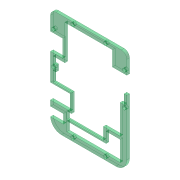
# Autodesk Inventor part: beagle_spacer_top
Saved by Autodesk Inventor 2014 (Build 180170000, 170)
## iProperties
Created: 2013-06-20
Part Number: beagle_spacer_top
Document SubType Name: Modeling
Designer: Administrator
Density: 1 g/cm^3
Mass: 28.363 g
Surface Area: 163.397 cm^2
Volume: 28.363 cm^3
Material: Generic
Appearance: Clear - Green 1
Author: Administrator
Autodesk Inventor part; units mm, degrees
ref_plane "YZ Plane" through (0, 0, 0) normal (1, 0, 0) x (0, 1, 0)
ref_plane "XZ Plane" through (0, 0, 0) normal (0, 1, 0) x (-1, 0, 0)
ref_plane "XY Plane" through (0, 0, 0) normal (0, 0, 1) x (1, 0, 0)
sketch "Sketch1" plane through (0, 0, 0) normal (0, 0, 1) x (1, 0, 0)
  line L0 (9.8795, 48.1994) -> (9.8795, -53.4006)
  line L1 (16.2295, 54.5494) -> (92.4295, 54.5494)
  line L2 (98.7795, 48.1994) -> (98.7795, -53.4006)
  line L3 (22.5795, -66.1006) -> (86.0795, -66.1006)
  arc A0 (9.8795, -53.4006) -> (22.5795, -66.1006) centre (22.5795, -53.4006) ccw
  arc A1 (16.2295, 54.5494) -> (9.8795, 48.1994) centre (16.2295, 48.1994) ccw
  arc A2 (98.7795, 48.1994) -> (92.4295, 54.5494) centre (92.4295, 48.1994) ccw
  arc A3 (86.0795, -66.1006) -> (98.7795, -53.4006) centre (86.0795, -53.4006) ccw
  point P0 (0, 0)
  dimension "d0" = 12.7
  dimension "d1" = 6.35
  dimension "d2" = 120.65
  dimension "d3" = 88.9
  constraints: 8 end point, 8 point on circle, 8 tangent, 4 centre point, 2 equal radius, 1 horizontal, 1 vertical
  measures "d0" radius of A0
  measures "d1" radius of A1
  measures "d2" distance between parallel lines of L3 L1
  measures "d3" distance between parallel lines of L2 L0
extrude "Extrusion1" add sketch "Sketch1" along normal blind 3.175
sketch "Sketch2" plane through (0, 0, 3.175) normal (0, 0, 1) x (1, 0, 0)
  line L0 (9.8795, -53.4006) -> (9.8795, 48.1994) projected
  line L1 (98.7795, 48.1994) -> (98.7795, -53.4006) projected
  line L2 (16.2295, 54.5494) -> (92.4295, 54.5494) projected
  line L3 (26.6435, 49.4694) -> (82.0155, 49.4694)
  line L4 (82.0155, 49.4694) -> (82.0155, -1.3306)
  line L5 (82.0155, -1.3306) -> (26.6435, -1.3306)
  line L6 (26.6435, -1.3306) -> (26.6435, 49.4694)
  point P0 (0, 0)
  dimension "d13" = 16.764
  dimension "d14" = 16.764
  dimension "d15" = 5.08
  dimension "d16" = 55.88
  constraints: 8 end point
  measures "d13" distance between parallel lines of L0 L6
  measures "d14" distance between parallel lines of L1 L4
  measures "d15" distance between parallel lines of L2 L3
  measures "d16" distance between parallel lines of L5 L2
extrude "Extrusion2" cut sketch "Sketch2" against normal through all
sketch "Sketch3" plane through (0, 0, 3.175) normal (0, 0, 1) x (1, 0, 0)
  line L0 (9.8795, -53.4006) -> (9.8795, 48.1994) projected
  line L1 (86.0795, -66.1006) -> (22.5795, -66.1006) projected
  line L2 (9.8795, -19.4408) -> (32.7395, -19.4408)
  line L3 (32.7395, -19.4408) -> (32.7395, -37.2208)
  line L4 (32.7395, -37.2208) -> (9.8795, -37.2208)
  point P0 (0, 0)
  dimension "d20" = 28.8798
  dimension "d21" = 46.6598
  dimension "d22" = 22.86
  constraints: 6 end point, 2 point on line
  measures "d20" distance between parallel lines of L4 L1
  measures "d21" distance between parallel lines of L1 L2
  measures "d22" distance between parallel lines of L3 L0
extrude "Extrusion3" cut sketch "Sketch3" against normal through all
sketch "Sketch4" plane through (0, 0, 3.175) normal (0, 0, 1) x (1, 0, 0)
  line L0 (9.8795, -53.4006) -> (9.8795, -37.2208) projected
  arc A0 (9.8795, -53.4006) -> (22.5795, -66.1006) centre (22.5795, -53.4006) ccw projected
  line L1 (86.0795, -66.1006) -> (22.5795, -66.1006) projected
  line L2 (24.8655, -43.5708) -> (24.8655, -54.1626)
  line L3 (24.8655, -43.5708) -> (9.8795, -43.5708)
  line L4 (24.8655, -54.1626) -> (9.9024, -54.1626)
  point P0 (0, 0)
  dimension "d26" = 22.5298
  dimension "d27" = 14.986
  dimension "d28" = 11.938
  constraints: 6 end point, 1 horizontal, 1 point on circle, 1 point on line, 1 vertical
  measures "d26" distance between parallel lines of L1 L3
  measures "d27" distance between parallel lines of L0 L2
  measures "d28" distance between parallel lines of L1 L4
extrude "Extrusion4" cut sketch "Sketch4" against normal through all
sketch "Sketch5" plane through (0, 0, 3.175) normal (0, 0, 1) x (1, 0, 0)
  line L0 (86.0795, -66.1006) -> (22.5795, -66.1006) projected
  line L1 (9.8795, -19.4408) -> (9.8795, 48.1994) projected
  line L2 (9.8795, -43.5708) -> (9.8795, -37.2208) projected
  line L3 (28.9295, -2.1688) -> (91.1595, -2.1688)
  line L4 (91.1595, -2.1688) -> (91.1595, -11.5668)
  line L5 (91.1595, -11.5668) -> (28.9295, -11.5668)
  line L6 (28.9295, -11.5668) -> (28.9295, -2.1688)
  line L7 (28.9295, -50.4288) -> (91.1595, -50.4288)
  line L8 (91.1595, -50.4288) -> (91.1595, -59.8268)
  line L9 (91.1595, -59.8268) -> (28.9295, -59.8268)
  line L10 (28.9295, -59.8268) -> (28.9295, -50.4288)
  point P0 (0, 0)
  dimension "d31" = 54.5338
  dimension "d32" = 9.398
  dimension "d33" = 62.23
  dimension "d34" = 19.05
  dimension "d35" = 19.05
  dimension "d36" = 6.2738
  constraints: 16 end point, 2 equal length
  measures "d31" distance between parallel lines of L0 L5
  measures "d32" distance between parallel lines of L3 L5
  measures "d33" distance of L4.end L5.end
  measures "d34" distance between parallel lines of L1 L6
  measures "d35" distance between parallel lines of L2 L10
  measures "d36" distance between parallel lines of L9 L0
extrude "Extrusion5" cut sketch "Sketch5" against normal through all
sketch "Sketch6" plane through (0, 0, 3.175) normal (0, 0, 1) x (1, 0, 0)
  line L0 (74.6495, -11.5668) -> (28.9295, -11.5668)
  line L1 (28.9295, -50.4288) -> (74.6495, -50.4288)
  line L2 (74.6495, -50.4288) -> (74.6495, -11.5668)
  line L3 (28.9295, -59.8268) -> (28.9295, -50.4288) projected
  line L4 (28.9295, -11.5668) -> (28.9295, -50.4288)
  line L5 (28.9295, -47.2538) -> (71.4745, -47.2538)
  line L6 (9.8795, -19.4408) -> (32.7395, -19.4408) projected
  line L7 (32.7395, -19.4408) -> (32.7395, -37.2208) projected
  line L8 (32.7395, -37.2208) -> (9.8795, -37.2208) projected
  line L9 (28.9295, -17.8533) -> (34.327, -17.8533)
  line L10 (34.327, -17.8533) -> (34.327, -38.8083)
  line L11 (34.327, -38.8083) -> (28.9295, -38.8083)
  line L12 (91.1595, -11.5668) -> (28.9295, -11.5668) projected
  line L13 (28.9295, -50.4288) -> (91.1595, -50.4288) projected
  line L14 (91.1595, -50.4288) -> (91.1595, -36.4588)
  line L15 (91.1595, -36.4588) -> (74.6495, -36.4588)
  line L16 (28.9295, -14.7418) -> (74.6495, -14.7418)
  line L17 (28.9295, -48.8413) -> (74.6495, -48.8413)
  line L18 (71.4745, -47.2538) -> (71.4745, -33.2838)
  line L19 (71.4745, -33.2838) -> (74.6495, -33.2838)
  line L20 (91.1595, -50.4288) -> (74.6495, -50.4288)
  line L21 (98.7795, 48.1994) -> (98.7795, -53.4006) projected
  line L22 (86.0795, -66.1006) -> (22.5795, -66.1006) projected
  point P0 (0, 0)
  dimension "d46" = 3.175
  dimension "d49" = 1.5875
  dimension "d50" = 1.5875
  dimension "d51" = 1.5875
  dimension "d55" = 3.175
  dimension "d57" = 1.5875
  dimension "d58" = 3.175
  dimension "d61" = 3.175
  dimension "d67" = 24.13
  dimension "d165" = 32.8168
  dimension "d166" = 13.97
  dimension "d167" = 29.6418
  dimension "d168" = 27.305
  constraints: 30 end point, 10 point on line, 4 vertical, 2 collinear
  measures "d46" distance between parallel lines of L1 L5
  measures "d49" distance between parallel lines of L8 L11
  measures "d50" distance between parallel lines of L10 L7
  measures "d51" distance between parallel lines of L6 L9
  measures "d55" distance between parallel lines of L12 L16
  measures "d57" distance between parallel lines of L1 L17
  measures "d58" distance between parallel lines of L15 L19
  measures "d61" distance between parallel lines of L2 L18
  measures "d67" distance between parallel lines of L21 L2
  measures "d165" distance between parallel lines of L22 L19
  measures "d166" distance of L13.end L14.end
  measures "d167" distance between parallel lines of L22 L15
  measures "d168" distance between parallel lines of L21 L18
extrude "Extrusion11" cut sketch "Sketch6" against normal through all contours L2 L19 L18 L5 L4 L11 L10 L9 L16 | L15 L14 L13 L2 | L2 L1 L4 L17
sketch "Sketch7" plane through (0, 0, 3.175) normal (0, 0, 1) x (1, 0, 0)
  line L0 (74.6495, -14.7418) -> (74.6495, -33.2838) projected
  line L1 (74.6495, -14.7418) -> (80.9995, -14.7418)
  line L2 (80.9995, -14.7418) -> (80.9995, -33.2838)
  line L3 (80.9995, -33.2838) -> (74.6495, -33.2838)
  point P0 (0, 0)
  dimension "d64" = 6.35
  constraints: 6 end point, 2 horizontal
  measures "d64" distance between parallel lines of L2 L0
extrude "Extrusion12" cut sketch "Sketch7" against normal through all
sketch "Sketch8" plane through (0, 0, 3.175) normal (0, 0, 1) x (1, 0, 0)
  line L0 (86.0795, -66.1006) -> (22.5795, -66.1006) projected
  line L1 (98.7795, 48.1994) -> (98.7795, -53.4006) projected
  line L2 (16.2295, 54.5494) -> (92.4295, 54.5494) projected
  line L3 (9.8795, -19.4408) -> (9.8795, 48.1994) projected
  line L4 (9.8795, -43.5708) -> (9.8795, -37.2208) projected
  line L5 (36.2694, 53.1397) -> (37.2593, 51.4252)
  line L6 (37.2593, 51.4252) -> (36.2694, 49.7107)
  line L7 (36.2694, 49.7107) -> (34.2897, 49.7107)
  line L8 (34.2897, 49.7107) -> (33.2998, 51.4252)
  line L9 (33.2998, 51.4252) -> (34.2897, 53.1397)
  line L10 (34.2897, 53.1397) -> (36.2694, 53.1397)
  line L11 (37.2593, -62.9764) -> (36.2694, -64.6909)
  line L12 (36.2694, -64.6909) -> (34.2897, -64.6909)
  line L13 (34.2897, -64.6909) -> (33.2998, -62.9764)
  line L14 (33.2998, -62.9764) -> (34.2897, -61.2619)
  line L15 (34.2897, -61.2619) -> (36.2694, -61.2619)
  line L16 (36.2694, -61.2619) -> (37.2593, -62.9764)
  line L17 (74.3694, -64.6909) -> (72.3897, -64.6909)
  line L18 (72.3897, -64.6909) -> (71.3998, -62.9764)
  line L19 (71.3998, -62.9764) -> (72.3897, -61.2619)
  line L20 (72.3897, -61.2619) -> (74.3694, -61.2619)
  line L21 (74.3694, -61.2619) -> (75.3593, -62.9764)
  line L22 (75.3593, -62.9764) -> (74.3694, -64.6909)
  line L23 (74.3694, 53.1397) -> (75.3593, 51.4252)
  line L24 (75.3593, 51.4252) -> (74.3694, 49.7107)
  line L25 (74.3694, 49.7107) -> (72.3897, 49.7107)
  line L26 (72.3897, 49.7107) -> (71.3998, 51.4252)
  line L27 (71.3998, 51.4252) -> (72.3897, 53.1397)
  line L28 (72.3897, 53.1397) -> (74.3694, 53.1397)
  line L29 (13.0037, 33.5197) -> (11.2892, 34.5095)
  line L30 (11.2892, 34.5095) -> (11.2892, 36.4893)
  line L31 (11.2892, 36.4893) -> (13.0037, 37.4791)
  line L32 (13.0037, 37.4791) -> (14.7182, 36.4893)
  line L33 (14.7182, 36.4893) -> (14.7182, 34.5095)
  line L34 (14.7182, 34.5095) -> (13.0037, 33.5197)
  line L35 (13.0037, -4.5803) -> (11.2892, -3.5905)
  line L36 (11.2892, -3.5905) -> (11.2892, -1.6107)
  line L37 (11.2892, -1.6107) -> (13.0037, -0.6209)
  line L38 (13.0037, -0.6209) -> (14.7182, -1.6107)
  line L39 (14.7182, -1.6107) -> (14.7182, -3.5905)
  line L40 (14.7182, -3.5905) -> (13.0037, -4.5803)
  line L41 (95.6553, 33.5197) -> (93.9408, 34.5095)
  line L42 (93.9408, 34.5095) -> (93.9408, 36.4893)
  line L43 (93.9408, 36.4893) -> (95.6553, 37.4791)
  line L44 (95.6553, 37.4791) -> (97.3698, 36.4893)
  line L45 (97.3698, 36.4893) -> (97.3698, 34.5095)
  line L46 (97.3698, 34.5095) -> (95.6553, 33.5197)
  line L47 (97.3698, -1.6107) -> (97.3698, -3.5905)
  line L48 (97.3698, -3.5905) -> (95.6553, -4.5803)
  line L49 (95.6553, -4.5803) -> (93.9408, -3.5905)
  line L50 (93.9408, -3.5905) -> (93.9408, -1.6107)
  line L51 (93.9408, -1.6107) -> (95.6553, -0.6209)
  line L52 (95.6553, -0.6209) -> (97.3698, -1.6107)
  point P0 (0, 0)
  point P1 (35.2795, 51.4252)
  point P2 (35.2795, -62.9764)
  point P3 (73.3795, -62.9764)
  point P4 (73.3795, 51.4252)
  point P5 (13.0037, 35.4994)
  point P6 (13.0037, -2.6006)
  point P7 (95.6553, 35.4994)
  point P8 (95.6553, -2.6006)
  dimension "d68" = 3.429
  dimension "d70" = 3.429
  dimension "d73" = 3.429
  dimension "d75" = 25.4
  dimension "d76" = 25.4
  dimension "d77" = 25.4
  dimension "d78" = 3.429
  dimension "d80" = 25.4
  dimension "d81" = 38.1
  dimension "d84" = 38.1
  dimension "d87" = 19.05
  dimension "d89" = 117.5258
  dimension "d90" = 101.6
  dimension "d91" = 63.5
  dimension "d92" = 85.7758
  dimension "d93" = 63.5
  dimension "d96" = 3.1242
  dimension "d97" = 3.1242
  dimension "d98" = 3.1242
  dimension "d99" = 3.1242
  constraints: 96 end point, 4 equal length, 4 horizontal, 4 vertical, 3 horizontal alignment, 2 vertical alignment, 104 other
  measures "d68" distance between parallel lines of L7 L10
  measures "d70" distance between parallel lines of L12 L15
  measures "d73" distance between parallel lines of L17 L20
  measures "d75" distance from line of L4 point (35.28, -62.976)
  measures "d76" distance from line of L1 point (73.38, -62.976)
  measures "d77" distance from line of L3 point (35.28, 51.425)
  measures "d78" distance between parallel lines of L25 L28
  measures "d80" distance from line of L1 point (73.38, 51.425)
  measures "d81" distance of point (13.004, -2.601) point (13.004, 35.499)
  measures "d84" distance of point (95.655, -2.601) point (95.655, 35.499)
  measures "d87" distance from line of L2 point (13.004, 35.499)
  measures "d89" distance from line of L0 point (35.28, 51.425)
  measures "d90" distance from line of L0 point (13.004, 35.499)
  measures "d91" distance from line of L0 point (13.004, -2.601)
  measures "d92" distance from line of L3 point (95.655, -2.601)
  measures "d93" distance from line of L3 point (73.38, 51.425)
  measures "d96" distance from line of L2 point (35.28, 51.425)
  measures "d97" distance from line of L3 point (13.004, 35.499)
  measures "d98" distance from line of L1 point (95.655, 35.499)
  measures "d99" distance from line of L0 point (35.28, -62.976)
extrude "Extrusion13" cut sketch "Sketch8" against normal through all
sketch "Sketch9" plane through (0, 0, 3.175) normal (0, 0, 1) x (1, 0, 0)
  line L0 (11.2892, 34.5095) -> (11.2892, 36.4893) projected
  line L1 (9.8795, -19.4408) -> (9.8795, 48.1994) projected
  line L2 (26.6435, -1.3306) -> (26.6435, 49.4694) projected
  line L3 (9.8795, 32.11) -> (24.1035, 32.11)
  line L4 (24.1035, 32.11) -> (24.1035, 11.79)
  line L5 (24.1035, 11.79) -> (9.8795, 11.79)
  line L6 (86.0795, -66.1006) -> (22.5795, -66.1006) projected
  line L7 (98.7795, 48.1994) -> (98.7795, -53.4006) projected
  line L8 (13.9435, 32.11) -> (13.9435, 11.79) construction
  point P0 (13.0037, 33.5197)
  point P1 (0, 0)
  dimension "d100" = 20.32
  dimension "d101" = 1.4097
  dimension "d102" = 1.4097
  dimension "d103" = 2.54
  dimension "d106" = 77.8906
  dimension "d107" = 10.16
  dimension "d108" = 74.676
  constraints: 8 end point, 4 point on line
  measures "d100" distance between parallel lines of L5 L3
  measures "d101" distance between parallel lines of L1 L0
  measures "d102" distance from line of L3 point (13.004, 33.52)
  measures "d103" distance between parallel lines of L2 L4
  measures "d106" distance between parallel lines of L6 L5
  measures "d107" distance between parallel lines of L4 L8
  measures "d108" distance between parallel lines of L4 L7
extrude "Extrusion14" cut sketch "Sketch9" against normal through all
sketch "Sketch10" plane through (0, 0, 3.175) normal (0, 0, 1) x (1, 0, 0)
  line L0 (28.9295, -11.5668) -> (28.9295, -2.1688) projected
  line L1 (28.9295, -2.1688) -> (91.1595, -2.1688) projected
  line L2 (91.1595, -11.5668) -> (28.9295, -11.5668) projected
  line L3 (26.6435, -1.3306) -> (26.6435, 49.4694) projected
  line L4 (82.0155, -1.3306) -> (26.6435, -1.3306) projected
  line L5 (24.1035, 11.79) -> (9.8795, 11.79) projected
  line L6 (9.8795, -19.4408) -> (9.8795, 11.79) projected
  line L7 (9.8795, -19.4408) -> (32.7395, -19.4408) projected
  line L8 (28.9295, -17.8533) -> (28.9295, -14.7418) projected
  line L9 (28.9295, -14.7418) -> (80.9995, -14.7418) projected
  line L10 (11.2892, -3.5905) -> (11.2892, -1.6107) projected
  line L11 (14.7182, -1.6107) -> (14.7182, -3.5905) projected
  line L12 (26.6435, 8.6658) -> (13.0037, 8.6658)
  line L13 (13.0037, 8.6658) -> (13.0037, 0.7888)
  line L14 (13.0037, 0.7888) -> (16.1279, 0.7888)
  line L15 (16.1279, 0.7888) -> (16.1279, -5.99)
  line L16 (16.1279, -5.99) -> (13.0037, -5.99)
  line L17 (13.0037, -5.99) -> (13.0037, -19.4408)
  line L18 (28.9295, -17.8533) -> (13.0037, -17.8533)
  line L19 (82.0155, -1.3306) -> (82.0155, -2.1688)
  line L20 (80.9995, -14.7418) -> (80.9995, -11.5668)
  point P0 (13.0037, -4.5803)
  point P1 (13.0037, -0.6209)
  point P2 (0, 0)
  dimension "d110" = 1.4097
  dimension "d111" = 1.4097
  dimension "d113" = 1.4097
  dimension "d114" = 1.4097
  dimension "d115" = 3.1242
  dimension "d116" = 3.1242
  dimension "d117" = 3.1242
  constraints: 18 end point, 5 point on line, 3 horizontal, 2 vertical
  measures "d110" distance between parallel lines of L6 L10
  measures "d111" distance between parallel lines of L15 L11
  measures "d113" distance from line of L16 point (13.004, -4.58)
  measures "d114" distance from line of L14 point (13.004, -0.621)
  measures "d115" distance between parallel lines of L6 L17
  measures "d116" distance between parallel lines of L6 L13
  measures "d117" distance between parallel lines of L5 L12
extrude "Extrusion15" cut sketch "Sketch10" against normal through all
sketch "Sketch11" plane through (0, 0, 3.175) normal (0, 0, 1) x (1, 0, 0)
  line L0 (91.1595, -11.5668) -> (80.9995, -11.5668) projected
  line L1 (80.9995, -11.5668) -> (80.9995, -33.2838) projected
  line L2 (91.1595, -11.5668) -> (91.1595, -33.2838)
  line L3 (91.1595, -33.2838) -> (80.9995, -33.2838)
  point P0 (0, 0)
  constraints: 4 end point, 1 horizontal, 1 vertical
extrude "Extrusion16" cut sketch "Sketch11" against normal through all
sketch "Sketch13" plane through (0, 0, 0) normal (0, 0, -1) x (-1, 0, 0)
  line L0 (-91.1595, -33.2838) -> (-91.1595, -2.1688) projected
  line L1 (-91.1595, -2.1688) -> (-82.0155, -2.1688) projected
  line L2 (-82.0155, -2.1688) -> (-82.0155, 49.4694) projected
  line L3 (-82.0155, 49.4694) -> (-26.6435, 49.4694) projected
  line L4 (-26.6435, 49.4694) -> (-26.6435, 8.6658) projected
  line L5 (-26.6435, 8.6658) -> (-13.0037, 8.6658) projected
  line L6 (-13.0037, 8.6658) -> (-13.0037, 0.7888) projected
  line L7 (-13.0037, 0.7888) -> (-16.1279, 0.7888) projected
  line L8 (-16.1279, 0.7888) -> (-16.1279, -5.99) projected
  line L9 (-16.1279, -5.99) -> (-13.0037, -5.99) projected
  line L10 (-13.0037, -5.99) -> (-13.0037, -17.8533) projected
  line L11 (-13.0037, -17.8533) -> (-34.327, -17.8533) projected
  line L12 (-34.327, -17.8533) -> (-34.327, -38.8083) projected
  line L13 (-34.327, -38.8083) -> (-28.9295, -38.8083) projected
  line L14 (-28.9295, -38.8083) -> (-28.9295, -47.2538) projected
  line L15 (-28.9295, -47.2538) -> (-71.4745, -47.2538) projected
  line L16 (-71.4745, -47.2538) -> (-71.4745, -33.2838) projected
  line L17 (-71.4745, -33.2838) -> (-91.1595, -33.2838) projected
  line L18 (-24.1035, 32.11) -> (-9.8795, 32.11) projected
  line L19 (-9.8795, 48.1994) -> (-9.8795, 32.11) projected
  arc A0 (-9.8795, 48.1994) -> (-16.2295, 54.5494) centre (-16.2295, 48.1994) ccw projected
  line L20 (-92.4295, 54.5494) -> (-16.2295, 54.5494) projected
  arc A1 (-92.4295, 54.5494) -> (-98.7795, 48.1994) centre (-92.4295, 48.1994) ccw projected
  line L21 (-98.7795, -53.4006) -> (-98.7795, 48.1994) projected
  arc A2 (-98.7795, -53.4006) -> (-86.0795, -66.1006) centre (-86.0795, -53.4006) ccw projected
  line L22 (-22.5795, -66.1006) -> (-86.0795, -66.1006) projected
  arc A3 (-22.5795, -66.1006) -> (-9.9024, -54.1626) centre (-22.5795, -53.4006) ccw projected
  line L23 (-9.9024, -54.1626) -> (-24.8655, -54.1626) projected
  line L24 (-24.8655, -54.1626) -> (-24.8655, -43.5708) projected
  line L25 (-24.8655, -43.5708) -> (-9.8795, -43.5708) projected
  line L26 (-9.8795, -37.2208) -> (-9.8795, -43.5708) projected
  line L27 (-9.8795, -37.2208) -> (-32.7395, -37.2208) projected
  line L28 (-32.7395, -37.2208) -> (-32.7395, -19.4408) projected
  line L29 (-32.7395, -19.4408) -> (-9.8795, -19.4408) projected
  line L30 (-9.8795, 11.79) -> (-9.8795, -19.4408) projected
  line L31 (-9.8795, 11.79) -> (-24.1035, 11.79) projected
  line L32 (-24.1035, 11.79) -> (-24.1035, 32.11) projected
  line L33 (-74.3694, 53.1397) -> (-72.3897, 53.1397) projected
  line L34 (-72.3897, 53.1397) -> (-71.3998, 51.4252) projected
  line L35 (-71.3998, 51.4252) -> (-72.3897, 49.7107) projected
  line L36 (-72.3897, 49.7107) -> (-74.3694, 49.7107) projected
  line L37 (-74.3694, 49.7107) -> (-75.3593, 51.4252) projected
  line L38 (-75.3593, 51.4252) -> (-74.3694, 53.1397) projected
  line L39 (-36.2694, 53.1397) -> (-34.2897, 53.1397) projected
  line L40 (-34.2897, 53.1397) -> (-33.2998, 51.4252) projected
  line L41 (-33.2998, 51.4252) -> (-34.2897, 49.7107) projected
  line L42 (-34.2897, 49.7107) -> (-36.2694, 49.7107) projected
  line L43 (-36.2694, 49.7107) -> (-37.2593, 51.4252) projected
  line L44 (-37.2593, 51.4252) -> (-36.2694, 53.1397) projected
  line L45 (-13.0037, 33.5197) -> (-14.7182, 34.5095) projected
  line L46 (-14.7182, 34.5095) -> (-14.7182, 36.4893) projected
  line L47 (-14.7182, 36.4893) -> (-13.0037, 37.4791) projected
  line L48 (-13.0037, 37.4791) -> (-11.2892, 36.4893) projected
  line L49 (-11.2892, 36.4893) -> (-11.2892, 34.5095) projected
  line L50 (-11.2892, 34.5095) -> (-13.0037, 33.5197) projected
  line L51 (-13.0037, -4.5803) -> (-14.7182, -3.5905) projected
  line L52 (-14.7182, -3.5905) -> (-14.7182, -1.6107) projected
  line L53 (-14.7182, -1.6107) -> (-13.0037, -0.6209) projected
  line L54 (-13.0037, -0.6209) -> (-11.2892, -1.6107) projected
  line L55 (-11.2892, -1.6107) -> (-11.2892, -3.5905) projected
  line L56 (-11.2892, -3.5905) -> (-13.0037, -4.5803) projected
  line L57 (-95.6553, 33.5197) -> (-97.3698, 34.5095) projected
  line L58 (-97.3698, 34.5095) -> (-97.3698, 36.4893) projected
  line L59 (-97.3698, 36.4893) -> (-95.6553, 37.4791) projected
  line L60 (-95.6553, 37.4791) -> (-93.9408, 36.4893) projected
  line L61 (-93.9408, 36.4893) -> (-93.9408, 34.5095) projected
  line L62 (-93.9408, 34.5095) -> (-95.6553, 33.5197) projected
  line L63 (-74.3694, -64.6909) -> (-75.3593, -62.9764) projected
  line L64 (-75.3593, -62.9764) -> (-74.3694, -61.2619) projected
  line L65 (-74.3694, -61.2619) -> (-72.3897, -61.2619) projected
  line L66 (-72.3897, -61.2619) -> (-71.3998, -62.9764) projected
  line L67 (-71.3998, -62.9764) -> (-72.3897, -64.6909) projected
  line L68 (-72.3897, -64.6909) -> (-74.3694, -64.6909) projected
  line L69 (-37.2593, -62.9764) -> (-36.2694, -61.2619) projected
  line L70 (-36.2694, -61.2619) -> (-34.2897, -61.2619) projected
  line L71 (-34.2897, -61.2619) -> (-33.2998, -62.9764) projected
  line L72 (-33.2998, -62.9764) -> (-34.2897, -64.6909) projected
  line L73 (-34.2897, -64.6909) -> (-36.2694, -64.6909) projected
  line L74 (-36.2694, -64.6909) -> (-37.2593, -62.9764) projected
  line L75 (-97.3698, -1.6107) -> (-95.6553, -0.6209) projected
  line L76 (-95.6553, -0.6209) -> (-93.9408, -1.6107) projected
  line L77 (-93.9408, -1.6107) -> (-93.9408, -3.5905) projected
  line L78 (-93.9408, -3.5905) -> (-95.6553, -4.5803) projected
  line L79 (-95.6553, -4.5803) -> (-97.3698, -3.5905) projected
  line L80 (-97.3698, -3.5905) -> (-97.3698, -1.6107) projected
  line L81 (-28.9295, -48.8413) -> (-28.9295, -59.8268) projected
  line L82 (-28.9295, -59.8268) -> (-91.1595, -59.8268) projected
  line L83 (-91.1595, -59.8268) -> (-91.1595, -36.4588) projected
  line L84 (-91.1595, -36.4588) -> (-74.6495, -36.4588) projected
  line L85 (-74.6495, -36.4588) -> (-74.6495, -48.8413) projected
  line L86 (-74.6495, -48.8413) -> (-28.9295, -48.8413) projected
  point P0 (0, 0)
  dimension "d122" = 72.136
  dimension "d123" = 74.7664
  dimension "d124" = 85.7758
  dimension "d125" = 82.6516
  dimension "d126" = 64.4525
  dimension "d127" = 69.85
  dimension "d128" = 27.2923
  dimension "d129" = 48.2473
  dimension "d130" = 60.1106
  dimension "d131" = 66.8894
  dimension "d132" = 74.676
  dimension "d133" = 77.8906
  dimension "d134" = 98.2106
  dimension "d135" = 46.6598
  dimension "d136" = 66.04
  dimension "d137" = 28.8798
  dimension "d138" = 22.5298
  dimension "d139" = 11.938
  dimension "d140" = 16.764
  dimension "d141" = 7.62
  dimension "d142" = 63.9318
  dimension "d143" = 32.8168
  dimension "d144" = 29.6418
  dimension "d145" = 24.13
  dimension "d146" = 27.305
  dimension "d147" = 17.2593
  dimension "d148" = 18.8468
  dimension "d149" = 115.57
  measures "d122" distance between parallel lines of L4 L21
  measures "d123" distance between parallel lines of L22 L5
  measures "d124" distance between parallel lines of L6 L21
  measures "d125" distance between parallel lines of L8 L21
  measures "d126" distance between parallel lines of L21 L12
  measures "d127" distance between parallel lines of L21 L14
  measures "d128" distance between parallel lines of L13 L22
  measures "d129" distance between parallel lines of L22 L11
  measures "d130" distance between parallel lines of L22 L9
  measures "d131" distance between parallel lines of L7 L22
  measures "d132" distance between parallel lines of L21 L32
  measures "d133" distance between parallel lines of L22 L31
  measures "d134" distance between parallel lines of L22 L18
  measures "d135" distance between parallel lines of L22 L29
  measures "d136" distance between parallel lines of L28 L21
  measures "d137" distance between parallel lines of L22 L27
  measures "d138" distance between parallel lines of L22 L25
  measures "d139" distance between parallel lines of L23 L22
  measures "d140" distance between parallel lines of L2 L21
  measures "d141" distance between parallel lines of L21 L0
  measures "d142" distance between parallel lines of L22 L1
  measures "d143" distance between parallel lines of L22 L17
  measures "d144" distance between parallel lines of L22 L84
  measures "d145" distance between parallel lines of L21 L85
  measures "d146" distance between parallel lines of L21 L16
  measures "d147" distance between parallel lines of L22 L86
  measures "d148" distance between parallel lines of L22 L15
  measures "d149" distance between parallel lines of L22 L3
sketch "Sketch14" plane through (0, 0, 0) normal (0, 0, -1) x (-1, 0, 0)
  line L0 (-91.1595, -2.1688) -> (-82.0155, -2.1688) projected
  line L1 (-82.0155, -2.1688) -> (-82.0155, 49.4694) projected
  line L2 (-98.7795, -53.4006) -> (-98.7795, 48.1994) projected
  line L3 (-97.3698, 34.5095) -> (-97.3698, 36.4893) projected
  line L4 (-97.3698, -3.5905) -> (-97.3698, -1.6107) projected
  line L5 (-98.7795, 32.11) -> (-82.0155, 32.11)
  line L6 (-95.6553, 11.79) -> (-98.7795, 11.79)
  line L7 (-95.6553, 11.79) -> (-95.6553, 0.7888)
  line L8 (-95.6553, 0.7888) -> (-91.1595, 0.7888)
  line L9 (-91.1595, 0.7888) -> (-91.1595, -2.1688)
  point P0 (-95.6553, 33.5197)
  point P1 (-95.6553, -0.6209)
  point P2 (0, 0)
  dimension "d151" = 1.4097
  dimension "d152" = 1.4097
  dimension "d153" = 1.4097
  dimension "d155" = 20.32
  dimension "d156" = 1.4097
  constraints: 10 end point, 4 point on line, 2 horizontal, 1 vertical
  measures "d151" distance from line of point (-95.655, -0.621) L8
  measures "d152" distance between parallel lines of L2 L4
  measures "d153" distance between parallel lines of L2 L3
  measures "d155" distance between parallel lines of L6 L5
  measures "d156" distance from line of L5 point (-95.655, 33.52)
extrude "Extrusion17" cut sketch "Sketch14" against normal through all
sketch "Sketch15" plane through (0, 0, 0) normal (0, 0, -1) x (-1, 0, 0)
  line L0 (-95.6553, 11.79) -> (-98.7795, 11.79) projected
  line L1 (-98.7795, -53.4006) -> (-98.7795, 11.79) projected
  arc A0 (-98.7795, -53.4006) -> (-86.0795, -66.1006) centre (-86.0795, -53.4006) ccw projected
  line L2 (-22.5795, -66.1006) -> (-86.0795, -66.1006) projected
  arc A1 (-22.5795, -66.1006) -> (-9.9024, -54.1626) centre (-22.5795, -53.4006) ccw projected
  line L3 (-9.9024, -54.1626) -> (-24.8655, -54.1626) projected
  line L4 (-24.8655, -54.1626) -> (-24.8655, -43.5708) projected
  line L5 (-24.8655, -43.5708) -> (-9.8795, -43.5708) projected
  line L6 (-9.8795, -37.2208) -> (-9.8795, -43.5708) projected
  line L7 (-9.8795, -37.2208) -> (-32.7395, -37.2208) projected
  line L8 (-32.7395, -37.2208) -> (-32.7395, -19.4408) projected
  line L9 (-32.7395, -19.4408) -> (-9.8795, -19.4408) projected
  line L10 (-9.8795, 11.79) -> (-9.8795, -19.4408) projected
  line L11 (-9.8795, 11.79) -> (-24.1035, 11.79) projected
  line L12 (-24.1035, 11.79) -> (-24.1035, 32.11) projected
  line L13 (-24.1035, 32.11) -> (-9.8795, 32.11) projected
  line L14 (-9.8795, 48.1994) -> (-9.8795, 32.11) projected
  arc A2 (-9.8795, 48.1994) -> (-16.2295, 54.5494) centre (-16.2295, 48.1994) ccw projected
  line L15 (-92.4295, 54.5494) -> (-16.2295, 54.5494) projected
  arc A3 (-92.4295, 54.5494) -> (-98.7795, 48.1994) centre (-92.4295, 48.1994) ccw projected
  line L16 (-98.7795, 32.11) -> (-98.7795, 48.1994) projected
  line L17 (-98.7795, 32.11) -> (-82.0155, 32.11) projected
  line L18 (-82.0155, 32.11) -> (-82.0155, 49.4694) projected
  line L19 (-82.0155, 49.4694) -> (-26.6435, 49.4694) projected
  line L20 (-26.6435, 49.4694) -> (-26.6435, 8.6658) projected
  line L21 (-26.6435, 8.6658) -> (-13.0037, 8.6658) projected
  line L22 (-13.0037, 8.6658) -> (-13.0037, 0.7888) projected
  line L23 (-13.0037, 0.7888) -> (-16.1279, 0.7888) projected
  line L24 (-16.1279, 0.7888) -> (-16.1279, -5.99) projected
  line L25 (-16.1279, -5.99) -> (-13.0037, -5.99) projected
  line L26 (-13.0037, -5.99) -> (-13.0037, -17.8533) projected
  line L27 (-13.0037, -17.8533) -> (-34.327, -17.8533) projected
  line L28 (-34.327, -17.8533) -> (-34.327, -38.8083) projected
  line L29 (-34.327, -38.8083) -> (-28.9295, -38.8083) projected
  line L30 (-28.9295, -38.8083) -> (-28.9295, -47.2538) projected
  line L31 (-28.9295, -47.2538) -> (-71.4745, -47.2538) projected
  line L32 (-71.4745, -47.2538) -> (-71.4745, -33.2838) projected
  line L33 (-71.4745, -33.2838) -> (-91.1595, -33.2838) projected
  line L34 (-91.1595, -33.2838) -> (-91.1595, 0.7888) projected
  line L35 (-91.1595, 0.7888) -> (-95.6553, 0.7888) projected
  line L36 (-95.6553, 0.7888) -> (-95.6553, 11.79) projected
  line L37 (-74.3694, 53.1397) -> (-72.3897, 53.1397) projected
  line L38 (-72.3897, 53.1397) -> (-71.3998, 51.4252) projected
  line L39 (-71.3998, 51.4252) -> (-72.3897, 49.7107) projected
  line L40 (-72.3897, 49.7107) -> (-74.3694, 49.7107) projected
  line L41 (-74.3694, 49.7107) -> (-75.3593, 51.4252) projected
  line L42 (-75.3593, 51.4252) -> (-74.3694, 53.1397) projected
  line L43 (-36.2694, 53.1397) -> (-34.2897, 53.1397) projected
  line L44 (-34.2897, 53.1397) -> (-33.2998, 51.4252) projected
  line L45 (-33.2998, 51.4252) -> (-34.2897, 49.7107) projected
  line L46 (-34.2897, 49.7107) -> (-36.2694, 49.7107) projected
  line L47 (-36.2694, 49.7107) -> (-37.2593, 51.4252) projected
  line L48 (-37.2593, 51.4252) -> (-36.2694, 53.1397) projected
  line L49 (-13.0037, 33.5197) -> (-14.7182, 34.5095) projected
  line L50 (-14.7182, 34.5095) -> (-14.7182, 36.4893) projected
  line L51 (-14.7182, 36.4893) -> (-13.0037, 37.4791) projected
  line L52 (-13.0037, 37.4791) -> (-11.2892, 36.4893) projected
  line L53 (-11.2892, 36.4893) -> (-11.2892, 34.5095) projected
  line L54 (-11.2892, 34.5095) -> (-13.0037, 33.5197) projected
  line L55 (-13.0037, -4.5803) -> (-14.7182, -3.5905) projected
  line L56 (-14.7182, -3.5905) -> (-14.7182, -1.6107) projected
  line L57 (-14.7182, -1.6107) -> (-13.0037, -0.6209) projected
  line L58 (-13.0037, -0.6209) -> (-11.2892, -1.6107) projected
  line L59 (-11.2892, -1.6107) -> (-11.2892, -3.5905) projected
  line L60 (-11.2892, -3.5905) -> (-13.0037, -4.5803) projected
  line L61 (-95.6553, 33.5197) -> (-97.3698, 34.5095) projected
  line L62 (-97.3698, 34.5095) -> (-97.3698, 36.4893) projected
  line L63 (-97.3698, 36.4893) -> (-95.6553, 37.4791) projected
  line L64 (-95.6553, 37.4791) -> (-93.9408, 36.4893) projected
  line L65 (-93.9408, 36.4893) -> (-93.9408, 34.5095) projected
  line L66 (-93.9408, 34.5095) -> (-95.6553, 33.5197) projected
  line L67 (-74.3694, -64.6909) -> (-75.3593, -62.9764) projected
  line L68 (-75.3593, -62.9764) -> (-74.3694, -61.2619) projected
  line L69 (-74.3694, -61.2619) -> (-72.3897, -61.2619) projected
  line L70 (-72.3897, -61.2619) -> (-71.3998, -62.9764) projected
  line L71 (-71.3998, -62.9764) -> (-72.3897, -64.6909) projected
  line L72 (-72.3897, -64.6909) -> (-74.3694, -64.6909) projected
  line L73 (-37.2593, -62.9764) -> (-36.2694, -61.2619) projected
  line L74 (-36.2694, -61.2619) -> (-34.2897, -61.2619) projected
  line L75 (-34.2897, -61.2619) -> (-33.2998, -62.9764) projected
  line L76 (-33.2998, -62.9764) -> (-34.2897, -64.6909) projected
  line L77 (-34.2897, -64.6909) -> (-36.2694, -64.6909) projected
  line L78 (-36.2694, -64.6909) -> (-37.2593, -62.9764) projected
  line L79 (-97.3698, -1.6107) -> (-95.6553, -0.6209) projected
  line L80 (-95.6553, -0.6209) -> (-93.9408, -1.6107) projected
  line L81 (-93.9408, -1.6107) -> (-93.9408, -3.5905) projected
  line L82 (-93.9408, -3.5905) -> (-95.6553, -4.5803) projected
  line L83 (-95.6553, -4.5803) -> (-97.3698, -3.5905) projected
  line L84 (-97.3698, -3.5905) -> (-97.3698, -1.6107) projected
  line L85 (-28.9295, -48.8413) -> (-28.9295, -59.8268) projected
  line L86 (-28.9295, -59.8268) -> (-91.1595, -59.8268) projected
  line L87 (-91.1595, -59.8268) -> (-91.1595, -36.4588) projected
  line L88 (-91.1595, -36.4588) -> (-74.6495, -36.4588) projected
  line L89 (-74.6495, -36.4588) -> (-74.6495, -48.8413) projected
  line L90 (-74.6495, -48.8413) -> (-28.9295, -48.8413) projected
  point P0 (0, 0)
  dimension "d159" = 98.2106
  dimension "d160" = 16.764
  dimension "d161" = 77.8906
  dimension "d162" = 3.1242
  dimension "d163" = 66.8894
  measures "d159" distance between parallel lines of L2 L17
  measures "d160" distance between parallel lines of L16 L18
  measures "d161" distance between parallel lines of L2 L0
  measures "d162" distance between parallel lines of L1 L36
  measures "d163" distance between parallel lines of L2 L35
equation "\"d14\" = d13"
equation "\"d35\" = d34"
equation "\"d102\" = d101"
equation "\"d111\" = d110"
equation "\"d113\" = d110"
equation "\"d114\" = d110"
body "Solid1"
